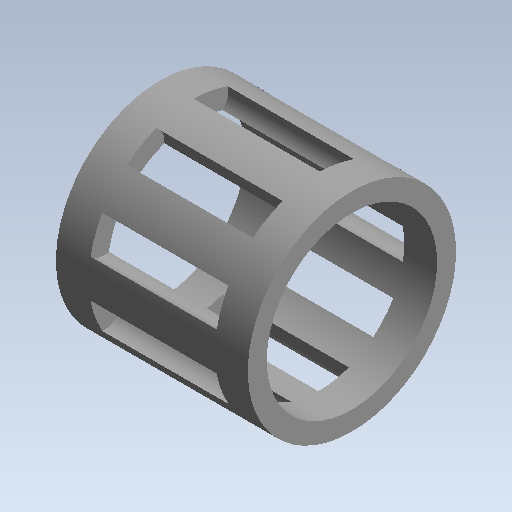
# Autodesk Inventor part: HK0609FMCA
Saved by Autodesk Inventor 2021.3 (Build 253353010, 353A)
## iProperties
Part Number: HK0609FMCA
Material: 一般
Catalog Web Link: www.cadenas.de
Description: Needle Roller Shell Bearings open-ended CA-
Vendor: NTN
Document SubType Name: Modeling
Designer: partserver
Manufacturer: NTN
Mass: 0.0858195 g
Surface Area: 3.66945 cm^2
Volume: 0.0858195 cm^3
Density: 1 g/cm^3
Appearance: PSOLRGB-192-192-192
Category: PARTsolutions
Company: NTN
PSOL_IDENT_0: {$CADENAS_DATA\23d-libs\ntn\needle_roler_bearings\needle_roller_shell_bearings_open_ended_ca.prj},19
PSOL_IDENT_1: 6 {VTYP=3D},{NB=HK0609FMCA},{LINA=HK0609FMCA},{NN=Needle Roller Shell Bearings open-ended CA},{DATE=
PSOL_IDENT_2: 23.10.2020 01:12:35},{GEOMDATE=20.04.2020 08:33:10},{VERSION=},{LINEID=40},{WBVAR=},{WBNUMERIC=}  {N
PSOL_IDENT_3: B=HK0609FMCA},{LINA=HK0609FMCA},{KT=DUMMY},{FW=6},{D=10.0},{C=9},{ORDER=HK0609FM},{CR=2920},{COR=259
PSOL_IDENT_4: 0},{CRF=298},{CORF=264},{LSG=25000},{LSO=37000},{MASS=0.0022},{IT=-},{RT=1.6},{VER=1},{T=0.500},{DW=
PSOL_IDENT_5: 1.500},{LW=5.000},{NR=9.000},{CID=6.750},{CD=8.250},{CW=7.600},{SD=6.300}
NB: HK0609FMCA
NN: Needle Roller Shell Bearings open-ended CA
NBSYN: $ORDER.CA
LINA: HK0609FMCA
CATALOG: NTN Corporation
FW: 6
D: 10
C: 9
ORDER: HK0609FM
CR: 2920
COR: 2590
CRF: 298
CORF: 264
LSG: 25000
LSO: 37000
MASS: 0.0022
IT: -
RT: 1.6
VER: 1
SUPPLIER: NTN
ARTICLENO: HK0609FMCA
BOMINFO: HK0609FMCA
CREATOR: CADENAS GmbH
Title: HK0609FMCA
Author: Cadenas PARTsolutions
Autodesk Inventor part; units mm, degrees
note: some values were not read from the file. Chosen so that the rebuilt part matches the saved one: pattern direction of "Circular Pattern1".
sketch "Sketch_1" plane through (0, 0, 0) normal (0, 0, 1) x (1, 0, 0)
  line L0 (8.3, 0) -> (0.7, 0)
  line L1 (0.7, 3.375) -> (8.3, 3.375)
  line L2 (8.3, 3.375) -> (8.3, 4.125)
  line L3 (8.3, 4.125) -> (0.7, 4.125)
  line L4 (0.7, 4.125) -> (0.7, 3.375)
  constraints: 10 end point
revolve "Revolution1" add sketch "Sketch_1" angle 360 about axis through (8.3, 0, 0) along (1, 0, 0)
sketch "Sketch_2" plane through (0, 0, 0) normal (0, 0, 1) x (1, 0, 0)
  line L0 (7, 3.75) -> (2, 3.75)
  line L1 (2, 3.75) -> (2, 4.5)
  line L2 (2, 4.5) -> (7, 4.5)
  line L3 (7, 4.5) -> (7, 3.75)
  line L4 (7, 3.75) -> (2, 3.75)
  constraints: 10 end point
revolve "Revolution2" cut sketch "Sketch_2" angle 360 about axis through (7, 3.75, 0) along (1, 0, 0)
pattern_circular "Circular Pattern1" count 9 over 360 about axis through (4.5, 0, 0) along (1, 0, 0) of "Revolution2"
ref_plane "IP_1_XY" through (4.5, 0, 0) normal (1, 0, 0) x (0, 0, -1)
ref_plane "IP_1_YZ" through (4.5, 0, 0) normal (0, 0, -1) x (0, 1, 0)
ref_plane "IP_1_ZX" through (4.5, 0, 0) normal (0, 1, 0) x (1, 0, 0)
ref_plane "IP_3_1_XY" through (4.5, 3.75, 0) normal (1, 0, 0) x (0, 0, -1)
ref_plane "IP_3_1_YZ" through (4.5, 3.75, 0) normal (0, 0, -1) x (0, 1, 0)
ref_plane "IP_3_1_ZX" through (4.5, 3.75, 0) normal (0, 1, 0) x (1, 0, 0)
ref_plane "IP_3_2_XY" through (4.5, 2.8727, 2.4105) normal (1, 0, 0) x (0, 0, -1)
ref_plane "IP_3_2_YZ" through (4.5, 2.8727, 2.4105) normal (0, 0, -1) x (0, 1, 0)
ref_plane "IP_3_2_ZX" through (4.5, 2.8727, 2.4105) normal (0, 1, 0) x (1, 0, 0)
ref_plane "IP_3_3_XY" through (4.5, 0.6512, 3.693) normal (1, 0, 0) x (0, 0, -1)
ref_plane "IP_3_3_YZ" through (4.5, 0.6512, 3.693) normal (0, 0, -1) x (0, 1, 0)
ref_plane "IP_3_3_ZX" through (4.5, 0.6512, 3.693) normal (0, 1, 0) x (1, 0, 0)
ref_plane "IP_3_4_XY" through (4.5, -1.875, 3.2476) normal (1, 0, 0) x (0, 0, -1)
ref_plane "IP_3_4_YZ" through (4.5, -1.875, 3.2476) normal (0, 0, -1) x (0, 1, 0)
ref_plane "IP_3_4_ZX" through (4.5, -1.875, 3.2476) normal (0, 1, 0) x (1, 0, 0)
ref_plane "IP_3_5_XY" through (4.5, -3.5238, 1.2826) normal (1, 0, 0) x (0, 0, -1)
ref_plane "IP_3_5_YZ" through (4.5, -3.5238, 1.2826) normal (0, 0, -1) x (0, 1, 0)
ref_plane "IP_3_5_ZX" through (4.5, -3.5238, 1.2826) normal (0, 1, 0) x (1, 0, 0)
ref_plane "IP_3_6_XY" through (4.5, -3.5238, -1.2826) normal (1, 0, 0) x (0, 0, -1)
ref_plane "IP_3_6_YZ" through (4.5, -3.5238, -1.2826) normal (0, 0, -1) x (0, 1, 0)
ref_plane "IP_3_6_ZX" through (4.5, -3.5238, -1.2826) normal (0, 1, 0) x (1, 0, 0)
ref_plane "IP_3_7_XY" through (4.5, -1.875, -3.2476) normal (1, 0, 0) x (0, 0, -1)
ref_plane "IP_3_7_YZ" through (4.5, -1.875, -3.2476) normal (0, 0, -1) x (0, 1, 0)
ref_plane "IP_3_7_ZX" through (4.5, -1.875, -3.2476) normal (0, 1, 0) x (1, 0, 0)
ref_plane "IP_3_8_XY" through (4.5, 0.6512, -3.693) normal (1, 0, 0) x (0, 0, -1)
ref_plane "IP_3_8_YZ" through (4.5, 0.6512, -3.693) normal (0, 0, -1) x (0, 1, 0)
ref_plane "IP_3_8_ZX" through (4.5, 0.6512, -3.693) normal (0, 1, 0) x (1, 0, 0)
ref_plane "IP_3_9_XY" through (4.5, 2.8727, -2.4105) normal (1, 0, 0) x (0, 0, -1)
ref_plane "IP_3_9_YZ" through (4.5, 2.8727, -2.4105) normal (0, 0, -1) x (0, 1, 0)
ref_plane "IP_3_9_ZX" through (4.5, 2.8727, -2.4105) normal (0, 1, 0) x (1, 0, 0)
body "Solid1"
